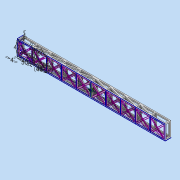
# Autodesk Inventor part: hashi1shado
Saved by Autodesk Inventor 2022 (Build 260153000, 153)
## iProperties
Created: 2024-05-14
Part Number: hashi1shado
Material: 一般
Document SubType Name: Modeling
Designer: ktamu
Density: 1 g/cm^3
Appearance: 既定
Mass: 75.4631 g
Surface Area: 713.328 cm^2
Volume: 75.4631 cm^3
Author: ktamu
Autodesk Inventor part; units mm, degrees
ref_plane "YZ Plane" through (0, 0, 0) normal (1, 0, 0) x (0, 1, 0)
ref_plane "XZ Plane" through (0, 0, 0) normal (0, 1, 0) x (-1, 0, 0)
ref_plane "XY Plane" through (0, 0, 0) normal (0, 0, 1) x (1, 0, 0)
sketch "スケッチ2" plane through (0, 0, 0) normal (1, 0, 0) x (0, 1, 0)
  line L0 (25, 10) -> (-25, 10)
  line L1 (-25, 10) -> (-25, -10)
  line L2 (-25, -10) -> (25, -10)
  line L3 (25, -10) -> (25, 10)
  line L4 (25, 10) -> (-25, -10) construction
  line L5 (-25, 10) -> (25, -10) construction
  point P0 (0, 0)
  dimension "d4" = 50
  dimension "d5" = 20
  constraints: 12 end point, 2 midpoint, 2 parallel, 1 horizontal, 1 perpendicular
  measures "d4" distance of L2.end L1.end
  measures "d5" distance of L1.end L0.end
sketch "スケッチ2 outline for 押し出し2" plane through (0, 0, 0) normal (1, 0, 0) x (0, 1, 0)
  line L0 (25, 10) -> (-25, 10)
  line L1 (25, -10) -> (25, 10)
  line L2 (-25, -10) -> (25, -10)
  line L3 (-25, 10) -> (-25, -10)
extrude "押し出し2" add sketch "スケッチ2 outline for 押し出し2" along normal mid plane 500
sketch "スケッチ3" plane through (-250, -25, 10) normal (0, 0, 1) x (1, 0, 0)
  circle A0 centre (250, 25) radius 5
  dimension "d8" = 10
  constraints: 1 centre point, 1 coincident
  measures "d8" diameter of A0
sketch "スケッチ3 outline for 押し出し3" plane through (-250, -25, 10) normal (0, 0, 1) x (1, 0, 0)
  circle A0 centre (250, 25) radius 5
extrude "押し出し3" add sketch "スケッチ3 outline for 押し出し3" along normal blind 2
sketch "SCfront" plane through (-250, -25, 10) normal (0, -1, 0) x (1, 0, 0)
  line L0 (0, -20) -> (500, -20)
  line L1 (500, 0) -> (500, -20)
  line L2 (500, 0) -> (0, 0)
  line L3 (0, -20) -> (0, 0)
  line L4 (0, 0) -> (500, 0)
  line L5 (500, 0) -> (500, -20)
  line L6 (500, -20) -> (0, -20)
  line L7 (0, -20) -> (0, 0)
  line L8 (0, 0) -> (500, -20) construction
  line L9 (500, 0) -> (0, -20) construction
  line L10 (0, 0) -> (500, 0)
  line L11 (0, -20) -> (500, -20)
  line L12 (0, 0) -> (50, 0)
  line L13 (50, 0) -> (50, -20)
  line L14 (50, -20) -> (0, -20)
  line L15 (0, -20) -> (0, 0)
  line L16 (100, 0) -> (100, -20)
  line L17 (150, 0) -> (150, -20)
  line L18 (200, 0) -> (200, -20)
  line L19 (250, 0) -> (250, -20)
  line L20 (450, 0) -> (450, -20)
  line L21 (400, 0) -> (400, -20)
  line L22 (350, 0) -> (350, -20)
  line L23 (300, 0) -> (300, -20)
  line L24 (0, 0) -> (0, -20)
  line L25 (0, 0) -> (50, -20)
  line L26 (0, -20) -> (50, 0) construction
  line L27 (50, 0) -> (100, -20)
  line L28 (100, 0) -> (50, -20)
  line L29 (52, -4) -> (98, -4)
  line L30 (98, -4) -> (98, -16)
  line L31 (98, -16) -> (52, -16)
  line L32 (52, -16) -> (52, -4)
  line L33 (75, -10) -> (98, -16) construction
  line L34 (98, -4) -> (52, -16) construction
  line L35 (102, -4) -> (148, -4)
  line L36 (102, -16) -> (102, -4)
  line L37 (148, -16) -> (102, -16)
  line L38 (148, -4) -> (148, -16)
  line L39 (152, -4) -> (198, -4)
  line L40 (152, -16) -> (152, -4)
  line L41 (198, -16) -> (152, -16)
  line L42 (198, -4) -> (198, -16)
  line L43 (202, -4) -> (248, -4)
  line L44 (202, -16) -> (202, -4)
  line L45 (248, -16) -> (202, -16)
  line L46 (248, -4) -> (248, -16)
  line L47 (252, -4) -> (298, -4)
  line L48 (252, -16) -> (252, -4)
  line L49 (298, -16) -> (252, -16)
  line L50 (298, -4) -> (298, -16)
  line L51 (302, -4) -> (348, -4)
  line L52 (302, -16) -> (302, -4)
  line L53 (348, -16) -> (302, -16)
  line L54 (348, -4) -> (348, -16)
  line L55 (352, -4) -> (398, -4)
  line L56 (352, -16) -> (352, -4)
  line L57 (398, -16) -> (352, -16)
  line L58 (398, -4) -> (398, -16)
  line L59 (402, -4) -> (448, -4)
  line L60 (402, -16) -> (402, -4)
  line L61 (448, -16) -> (402, -16)
  line L62 (448, -4) -> (448, -16)
  line L63 (48, -4) -> (48, -16)
  line L64 (48, -4) -> (4, -4)
  line L65 (4, -4) -> (4, -16.342138)
  line L66 (4, -16.342138) -> (48, -16.342138)
  line L67 (48, -16.342138) -> (48, -4)
  line L68 (452, -4) -> (452, -16)
  line L69 (452, -4) -> (496, -4)
  line L70 (496, -4) -> (496, -16.342138)
  line L71 (496, -16.342138) -> (452, -16.342138)
  line L72 (11.405237, -4) -> (48, -14.264946)
  line L73 (4, -6.077192) -> (40.594763, -16.342138)
  line L74 (488.594763, -4) -> (452, -14.264946)
  line L75 (496, -6.077192) -> (459.405237, -16.342138)
  line L76 (52, -4) -> (75, -10)
  line L77 (52, -6.066933) -> (90.076757, -16)
  line L78 (52.504844, -2.064765) -> (52.665247, -2.10661)
  line L79 (59.923243, -4) -> (98, -13.933067)
  line L80 (109.923243, -4) -> (148, -13.933067)
  line L81 (102, -6.066933) -> (140.076757, -16)
  line L82 (159.923243, -4) -> (198, -13.933067)
  line L83 (152, -6.066933) -> (190.076757, -16)
  line L84 (209.923243, -4) -> (248, -13.933067)
  line L85 (202, -6.066933) -> (240.076757, -16)
  line L86 (448, -6.066933) -> (409.923243, -16)
  line L87 (440.076757, -4) -> (402, -13.933067)
  line L88 (390.076757, -4) -> (352, -13.933067)
  line L89 (398, -6.066933) -> (359.923243, -16)
  line L90 (340.076757, -4) -> (302, -13.933067)
  line L91 (348, -6.066933) -> (309.923243, -16)
  line L92 (290.076757, -4) -> (252, -13.933067)
  line L93 (298, -6.066933) -> (259.923243, -16)
  point P0 (250, -10)
  point P1 (440.076757, -4)
  point P2 (390.076757, -4)
  point P3 (340.076757, -4)
  point P4 (290.076757, -4)
  point P5 (209.923243, -4)
  point P6 (159.923243, -4)
  point P7 (109.923243, -4)
  point P8 (60.14392, -4.057568)
  point P9 (60, -4)
  point P10 (90, -16)
  point P11 (89.85608, -15.942432)
  point P12 (48, -14.264946)
  dimension "d12" = 50
  dimension "d15" = 50
  dimension "d20" = 46
  dimension "d21" = 12
  dimension "d24" = 50
  dimension "d29" = 4
  dimension "d30" = 4
  dimension "d33" = 4
  dimension "d37" = 2
  dimension "d40" = 50
  constraints: 174 end point, 33 symmetric about line, 11 parallel, 11 point on line, 7 horizontal, 5 midpoint, 4 perpendicular, 1 vertical, 86 other
  measures "d12" distance of L13.end L14.end
  measures "d15" distance of L12.end L16.start
  measures "d20" distance of L30.end L31.end
  measures "d21" distance of L29.end L30.end
  measures "d24" distance of L29.start L35.start
  measures "d29" distance between parallel lines of L32 L63
  measures "d30" distance between parallel lines of L65 L3
  measures "d33" distance between parallel lines of L12 L64
  measures "d37" distance between parallel lines of L76 L77
  measures "d40" distance of L79.start L80.start
sketch "SCfront outline for 押し出し4" plane through (-250, -25, 10) normal (0, -1, 0) x (1, 0, 0)
  line L0 (496, -6.077192) -> (459.405237, -16.342138)
  line L1 (496, -16.342138) -> (496, -6.077192)
  line L2 (459.405237, -16.342138) -> (496, -16.342138)
  line L3 (452, -14.264946) -> (488.594763, -4)
  line L4 (452, -4) -> (452, -14.264946)
  line L5 (488.594763, -4) -> (452, -4)
  line L6 (448, -6.066933) -> (409.923243, -16)
  line L7 (448, -16) -> (448, -6.066933)
  line L8 (409.923243, -16) -> (448, -16)
  line L9 (402, -13.933067) -> (440.076757, -4)
  line L10 (402, -4) -> (402, -13.933067)
  line L11 (440.076757, -4) -> (402, -4)
  line L12 (398, -6.066933) -> (359.923243, -16)
  line L13 (398, -16) -> (398, -6.066933)
  line L14 (359.923243, -16) -> (398, -16)
  line L15 (352, -13.933067) -> (390.076757, -4)
  line L16 (352, -4) -> (352, -13.933067)
  line L17 (390.076757, -4) -> (352, -4)
  line L18 (348, -6.066933) -> (309.923243, -16)
  line L19 (348, -16) -> (348, -6.066933)
  line L20 (309.923243, -16) -> (348, -16)
  line L21 (302, -13.933067) -> (340.076757, -4)
  line L22 (302, -4) -> (302, -13.933067)
  line L23 (340.076757, -4) -> (302, -4)
  line L24 (298, -6.066933) -> (259.923243, -16)
  line L25 (298, -16) -> (298, -6.066933)
  line L26 (259.923243, -16) -> (298, -16)
  line L27 (252, -13.933067) -> (290.076757, -4)
  line L28 (252, -4) -> (252, -13.933067)
  line L29 (290.076757, -4) -> (252, -4)
  line L30 (209.923243, -4) -> (248, -13.933067)
  line L31 (248, -4) -> (209.923243, -4)
  line L32 (248, -13.933067) -> (248, -4)
  line L33 (240.076757, -16) -> (202, -6.066933)
  line L34 (202, -16) -> (240.076757, -16)
  line L35 (202, -6.066933) -> (202, -16)
  line L36 (159.923243, -4) -> (198, -13.933067)
  line L37 (198, -4) -> (159.923243, -4)
  line L38 (198, -13.933067) -> (198, -4)
  line L39 (190.076757, -16) -> (152, -6.066933)
  line L40 (152, -16) -> (190.076757, -16)
  line L41 (152, -6.066933) -> (152, -16)
  line L42 (109.923243, -4) -> (148, -13.933067)
  line L43 (148, -4) -> (109.923243, -4)
  line L44 (148, -13.933067) -> (148, -4)
  line L45 (140.076757, -16) -> (102, -6.066933)
  line L46 (102, -16) -> (140.076757, -16)
  line L47 (102, -6.066933) -> (102, -16)
  line L48 (60.14392, -4.057568) -> (98, -13.933067)
  line L49 (60, -4) -> (60.14392, -4.057568)
  line L50 (98, -4) -> (60, -4)
  line L51 (98, -13.933067) -> (98, -4)
  line L52 (89.85608, -15.942432) -> (52, -6.066933)
  line L53 (90, -16) -> (89.85608, -15.942432)
  line L54 (52, -16) -> (90, -16)
  line L55 (52, -6.066933) -> (52, -16)
  line L56 (11.405237, -4) -> (48, -14.264946)
  line L57 (48, -4) -> (11.405237, -4)
  line L58 (48, -14.264946) -> (48, -4)
  line L59 (40.594763, -16.342138) -> (4, -6.077192)
  line L60 (4, -16.342138) -> (40.594763, -16.342138)
  line L61 (4, -6.077192) -> (4, -16.342138)
extrude "押し出し4" cut sketch "SCfront outline for 押し出し4" against normal through all
sketch "SCLeft" plane through (-250, 0, 0) normal (-1, 0, 0) x (0, 0, 1)
  line L0 (10, 25) -> (10, -25)
  line L1 (-10, 25) -> (10, 25)
  line L2 (10, 25) -> (10, -25)
  line L3 (10, -25) -> (-10, -25)
  line L4 (-10, -25) -> (-10, 25)
  line L5 (-10, 25) -> (10, -25) construction
  line L6 (10, 25) -> (-10, -25) construction
  line L7 (-6, 21) -> (6, 21)
  line L8 (6, 21) -> (6, -21)
  line L9 (6, -21) -> (-6, -21)
  line L10 (-6, -21) -> (-6, 21)
  line L11 (-6, 21) -> (-1.040016, 3.640055) construction
  line L12 (6, 21) -> (-6, -21) construction
  line L13 (7.415352, 0) -> (4.34275, 0)
  line L14 (2.080031, 0) -> (6, -13.71989)
  line L15 (-3.919969, 21) -> (0, 7.28011)
  line L16 (-6, 21) -> (-1.040016, 3.640055)
  line L17 (1.040016, -3.640055) -> (6, -21)
  line L18 (-6, 13.71989) -> (-2.080031, 0)
  line L19 (0, -7.28011) -> (3.919969, -21)
  line L20 (0, 7.28011) -> (3.919969, 21)
  line L21 (-6, -13.71989) -> (-2.080031, 0)
  line L22 (-3.919969, -21) -> (0, -7.28011)
  line L23 (2.080031, 0) -> (6, 13.71989)
  line L24 (10, -25) -> (-10, -25)
  line L25 (-10, -25) -> (-10, 25)
  line L26 (-10, 25) -> (10, 25)
  line L27 (10, 25) -> (10, -25)
  line L28 (6, 15) -> (-6, 15)
  line L29 (-6, 15) -> (-6, -15)
  line L30 (-6, -15) -> (6, -15)
  line L31 (6, -15) -> (6, 15)
  line L32 (6, 15) -> (-6, -15) construction
  line L33 (-6, 15) -> (6, -15) construction
  point P0 (0, 0)
  dimension "d47" = 12
  dimension "d48" = 42
  dimension "d96" = 4
  dimension "d97" = 4
  constraints: 58 end point, 10 parallel, 6 point on line, 5 midpoint, 4 horizontal, 4 symmetric about line, 3 perpendicular
  measures "d47" distance of L8.end L9.end
  measures "d48" distance of L7.end L8.end
  measures "d96" distance between parallel lines of L4 L29
  measures "d97" distance between parallel lines of L26 L7
sketch "SCLeft outline for 押し出し5left" plane through (-250, 0, 0) normal (-1, 0, 0) x (0, 0, 1)
  line L0 (-6, 21) -> (-6, -21)
  line L1 (6, 21) -> (-6, 21)
  line L2 (6, -21) -> (6, 21)
  line L3 (-6, -21) -> (6, -21)
extrude "押し出し5left" cut sketch "SCLeft outline for 押し出し5left" against normal through all
sketch "SCLeft outline for 押し出し6" plane through (-250, 0, 0) normal (-1, 0, 0) x (0, 0, 1)
  line L0 (2.080031, 0) -> (6, 13.71989)
  line L1 (6, -13.71989) -> (2.080031, 0)
  line L2 (6, -21) -> (6, -13.71989)
  line L3 (3.919969, -21) -> (6, -21)
  line L4 (0, -7.28011) -> (3.919969, -21)
  line L5 (-3.919969, -21) -> (0, -7.28011)
  line L6 (-6, -21) -> (-3.919969, -21)
  line L7 (-6, -13.71989) -> (-6, -21)
  line L8 (-2.080031, 0) -> (-6, -13.71989)
  line L9 (-6, 13.71989) -> (-2.080031, 0)
  line L10 (-6, 21) -> (-6, 13.71989)
  line L11 (-3.919969, 21) -> (-6, 21)
  line L12 (0, 7.28011) -> (-3.919969, 21)
  line L13 (3.919969, 21) -> (0, 7.28011)
  line L14 (6, 21) -> (3.919969, 21)
  line L15 (6, 13.71989) -> (6, 21)
extrude "押し出し6" add sketch "SCLeft outline for 押し出し6" against normal blind 4
mirror "ミラー1" about plane through (0, 0, 0) normal (1, 0, 0) of "押し出し6"
sketch "SCtop" plane through (-250, -25, 10) normal (0, 0, 1) x (1, 0, 0)
  circle A0 centre (250, 25) radius 5
  line L0 (500, 0) -> (0, 0)
  line L1 (500, 50) -> (500, 0)
  line L2 (0, 50) -> (500, 50)
  line L3 (0, 0) -> (0, 50)
  circle A1 centre (250, 25) radius 5
  line L4 (0, 0) -> (0, 50)
  line L5 (0, 50) -> (500, 0) construction
  line L6 (0, 0) -> (500, 0)
  line L7 (500, 50) -> (0, 0) construction
  line L8 (0, 50) -> (500, 50)
  line L9 (500, 50) -> (500, 0)
  line L10 (500, 0) -> (0, 0)
  line L11 (0, 0) -> (0, 50)
  line L12 (0, 50) -> (500, 0) construction
  line L13 (500, 50) -> (0, 0) construction
  line L14 (0, 50) -> (500, 50)
  line L15 (0, 50) -> (50, 50)
  line L16 (50, 50) -> (50, 0)
  line L17 (50, 0) -> (0, 0)
  line L18 (0, 0) -> (0, 50)
  line L19 (100, 50) -> (100, 0)
  line L20 (150, 50) -> (150, 0)
  line L21 (200, 50) -> (200, 0)
  line L22 (250, 50) -> (250, 0)
  line L23 (300, 50) -> (300, 0)
  line L24 (350, 50) -> (350, 0)
  line L25 (400, 50) -> (400, 0)
  line L26 (450, 50) -> (450, 0)
  line L27 (50, 50) -> (100, 0)
  line L28 (0, 50) -> (50, 0)
  line L29 (50, 50) -> (0, 0)
  line L30 (98, 4) -> (60.14392, 4)
  line L31 (52, 46) -> (98, 46)
  line L32 (98, 46) -> (98, 4)
  line L33 (98, 4) -> (52, 4)
  line L34 (52, 4) -> (52, 46)
  line L35 (4, 46) -> (48, 46)
  line L36 (48, 46) -> (48, 4)
  line L37 (48, 4) -> (4, 4)
  line L38 (4, 4) -> (4, 46)
  line L39 (6.828427, 46) -> (48.025843, 4.802584)
  line L40 (4, 43.171573) -> (43.171573, 4)
  line L41 (25, 25) -> (25, 18.621886)
  line L42 (98, 0) -> (98, 4)
  line L43 (53.475936, 44.652406) -> (98, 4)
  line L44 (52, 43.291755) -> (95.033826, 4)
  line L45 (54.966174, 46) -> (98, 6.708245)
  line L46 (98, 43.291755) -> (54.966174, 4)
  line L47 (92.274678, 40.772532) -> (53.475936, 5.347594)
  line L48 (95.033826, 46) -> (52, 6.708245)
  line L49 (50.144939, 5.014494) -> (50, 4.882159)
  line L50 (73.584326, 23.584326) -> (90.909091, 40.909091)
  line L51 (92.274678, 40.772532) -> (73.516913, 23.645877) construction
  line L52 (53.475936, 5.347594) -> (52, 4) construction
  line L53 (52, 46) -> (53.475936, 44.652406) construction
  line L54 (73.516913, 26.354123) -> (98, 4) construction
  line L55 (48, 46) -> (4, 4)
  line L56 (45.103446, 46) -> (4, 6.764892)
  line L57 (48, 43.235108) -> (6.896554, 4)
  line L58 (104.966174, 46) -> (148, 6.708245)
  line L59 (145.033826, 46) -> (102, 6.708245)
  line L60 (148, 43.291755) -> (104.966174, 4)
  line L61 (102, 43.291755) -> (145.033826, 4)
  line L62 (148, 46) -> (148, 4)
  line L63 (102, 46) -> (148, 46)
  line L64 (102, 4) -> (102, 46)
  line L65 (148, 4) -> (102, 4)
  line L66 (154.966174, 46) -> (198, 6.708245)
  line L67 (195.033826, 46) -> (152, 6.708245)
  line L68 (198, 43.291755) -> (154.966174, 4)
  line L69 (152, 43.291755) -> (195.033826, 4)
  line L70 (198, 46) -> (198, 4)
  line L71 (152, 46) -> (198, 46)
  line L72 (152, 4) -> (152, 46)
  line L73 (198, 4) -> (152, 4)
  line L74 (204.966174, 46) -> (248, 6.708245)
  line L75 (245.033826, 46) -> (202, 6.708245)
  line L76 (248, 43.291755) -> (204.966174, 4)
  line L77 (202, 43.291755) -> (245.033826, 4)
  line L78 (248, 46) -> (248, 4)
  line L79 (202, 46) -> (248, 46)
  line L80 (202, 4) -> (202, 46)
  line L81 (248, 4) -> (202, 4)
  line L82 (254.966174, 46) -> (298, 6.708245)
  line L83 (295.033826, 46) -> (252, 6.708245)
  line L84 (298, 43.291755) -> (254.966174, 4)
  line L85 (252, 43.291755) -> (295.033826, 4)
  line L86 (298, 46) -> (298, 4)
  line L87 (252, 46) -> (298, 46)
  line L88 (252, 4) -> (252, 46)
  line L89 (298, 4) -> (252, 4)
  line L90 (304.966174, 46) -> (348, 6.708245)
  line L91 (345.033826, 46) -> (302, 6.708245)
  line L92 (348, 43.291755) -> (304.966174, 4)
  line L93 (302, 43.291755) -> (345.033826, 4)
  line L94 (348, 46) -> (348, 4)
  line L95 (302, 46) -> (348, 46)
  line L96 (302, 4) -> (302, 46)
  line L97 (348, 4) -> (302, 4)
  line L98 (354.966174, 46) -> (398, 6.708245)
  line L99 (395.033826, 46) -> (352, 6.708245)
  line L100 (398, 43.291755) -> (354.966174, 4)
  line L101 (352, 43.291755) -> (395.033826, 4)
  line L102 (398, 46) -> (398, 4)
  line L103 (352, 46) -> (398, 46)
  line L104 (352, 4) -> (352, 46)
  line L105 (398, 4) -> (352, 4)
  line L106 (404.966174, 46) -> (448, 6.708245)
  line L107 (445.033826, 46) -> (402, 6.708245)
  line L108 (448, 43.291755) -> (404.966174, 4)
  line L109 (402, 43.291755) -> (445.033826, 4)
  line L110 (448, 46) -> (448, 4)
  line L111 (402, 46) -> (448, 46)
  line L112 (402, 4) -> (402, 46)
  line L113 (448, 4) -> (402, 4)
  line L114 (496, 46) -> (452, 46)
  line L115 (452, 46) -> (452, 4)
  line L116 (452, 4) -> (496, 4)
  line L117 (496, 4) -> (496, 46)
  line L118 (493.171573, 46) -> (451.974157, 4.802584)
  line L119 (496, 43.171573) -> (456.828427, 4)
  line L120 (454.896554, 46) -> (496, 6.764892)
  line L121 (452, 43.235108) -> (493.103446, 4)
  point P0 (75, 25)
  point P1 (123.516913, 26.354123)
  point P2 (123.584326, 23.584326)
  point P3 (123.516913, 23.645877)
  point P4 (173.516913, 26.354123)
  point P5 (173.584326, 23.584326)
  point P6 (173.516913, 23.645877)
  point P7 (223.516913, 26.354123)
  point P8 (223.584326, 23.584326)
  point P9 (223.516913, 23.645877)
  point P10 (273.516913, 26.354123)
  point P11 (273.584326, 23.584326)
  point P12 (273.516913, 23.645877)
  point P13 (323.516913, 26.354123)
  point P14 (323.584326, 23.584326)
  point P15 (323.516913, 23.645877)
  point P16 (373.516913, 26.354123)
  point P17 (373.584326, 23.584326)
  point P18 (373.516913, 23.645877)
  point P19 (423.516913, 26.354123)
  point P20 (423.584326, 23.584326)
  point P21 (423.516913, 23.645877)
  point P22 (474.544134, 21.715707)
  point P23 (477.373326, 24.544899)
  point P24 (474.479122, 27.307549)
  point P25 (452, 4.828427)
  point P26 (471.64993, 24.478357)
  point P27 (427.966174, 25)
  point P28 (425, 22.291755)
  point P29 (425, 27.708245)
  point P30 (375, 22.291755)
  point P31 (375, 27.708245)
  point P32 (422.033826, 25)
  point P33 (377.966174, 25)
  point P34 (372.033826, 25)
  point P35 (327.966174, 25)
  point P36 (325, 22.291755)
  point P37 (325, 27.708245)
  point P38 (322.033826, 25)
  point P39 (275, 22.291755)
  point P40 (277.966174, 25)
  point P41 (275, 27.708245)
  point P42 (252, 20.417424)
  point P43 (272.033826, 25)
  point P44 (252, 29.582576)
  point P45 (225, 22.291755)
  point P46 (248, 29.582576)
  point P47 (227.966174, 25)
  point P48 (248, 20.417424)
  point P49 (225, 27.708245)
  point P50 (222.033826, 25)
  point P51 (175, 22.291755)
  point P52 (177.966174, 25)
  point P53 (175, 27.708245)
  point P54 (172.033826, 25)
  point P55 (125, 22.291755)
  point P56 (127.966174, 25)
  point P57 (125, 27.708245)
  point P58 (122.033826, 25)
  point P59 (77.966174, 25)
  point P60 (75, 22.291755)
  point P61 (75, 27.708245)
  point P62 (72.033826, 25)
  point P63 (25.455866, 21.715707)
  point P64 (28.35007, 24.478357)
  point P65 (48, 4.828427)
  point P66 (22.626674, 24.544899)
  point P67 (25.520878, 27.307549)
  point P68 (76.483087, 26.354123)
  point P69 (75, 25)
  point P70 (75, 25)
  point P71 (75, 25)
  point P72 (75, 25)
  point P73 (75, 25)
  point P74 (75, 25)
  point P75 (96, 4)
  point P76 (73.516913, 23.645877)
  point P77 (73.516913, 26.354123)
  point P78 (73.584326, 26.415674)
  point P79 (76.415674, 26.415674)
  point P80 (76.483087, 23.645877)
  point P81 (76.415674, 23.584326)
  dimension "d55" = 50
  dimension "d56" = 50
  dimension "d59" = 50
  dimension "d64" = 46
  dimension "d65" = 42
  dimension "d66" = 44
  dimension "d67" = 42
  dimension "d68" = 4
  dimension "d69" = 4
  dimension "d76" = 2
  dimension "d77" = 2
  dimension "d80" = 50
  constraints: 226 end point, 97 point on line, 20 midpoint, 17 parallel, 12 symmetric about line, 6 horizontal, 5 perpendicular, 1 vertical, 185 other
  measures "d55" distance of L16.end L17.end
  measures "d56" distance of L15.end L16.end
  measures "d59" distance of L15.end L19.start
  measures "d64" distance of L30.start L33.end
  measures "d65" distance of L31.end L30.start
  measures "d66" distance of L36.end L37.end
  measures "d67" distance of L35.end L36.end
  measures "d68" distance between parallel lines of L2 L35
  measures "d69" distance between parallel lines of L34 L36
  measures "d76" distance between parallel lines of L55 L56
  measures "d77" distance between parallel lines of L55 L57
  measures "d80" distance of L45.start L58.start
sketch "SCtop outline for 押し出し7" plane through (-250, -25, 10) normal (0, 0, 1) x (1, 0, 0)
  line L0 (456.828427, 4) -> (493.103446, 4)
  line L1 (474.544134, 21.715707) -> (456.828427, 4)
  line L2 (493.103446, 4) -> (474.544134, 21.715707)
  line L3 (496, 6.764892) -> (496, 43.171573)
  line L4 (477.373326, 24.544899) -> (496, 6.764892)
  line L5 (496, 43.171573) -> (477.373326, 24.544899)
  line L6 (493.171573, 46) -> (454.896554, 46)
  line L7 (474.479122, 27.307549) -> (493.171573, 46)
  line L8 (454.896554, 46) -> (474.479122, 27.307549)
  line L9 (452, 43.235108) -> (452, 4.828427)
  line L10 (471.64993, 24.478357) -> (452, 43.235108)
  line L11 (452, 4.828427) -> (471.64993, 24.478357)
  line L12 (448, 6.708245) -> (448, 43.291755)
  line L13 (427.966174, 25) -> (448, 6.708245)
  line L14 (448, 43.291755) -> (427.966174, 25)
  line L15 (404.966174, 4) -> (445.033826, 4)
  line L16 (425, 22.291755) -> (404.966174, 4)
  line L17 (445.033826, 4) -> (425, 22.291755)
  line L18 (445.033826, 46) -> (404.966174, 46)
  line L19 (425, 27.708245) -> (445.033826, 46)
  line L20 (404.966174, 46) -> (425, 27.708245)
  line L21 (354.966174, 4) -> (395.033826, 4)
  line L22 (375, 22.291755) -> (354.966174, 4)
  line L23 (395.033826, 4) -> (375, 22.291755)
  line L24 (395.033826, 46) -> (354.966174, 46)
  line L25 (375, 27.708245) -> (395.033826, 46)
  line L26 (354.966174, 46) -> (375, 27.708245)
  line L27 (402, 43.291755) -> (402, 6.708245)
  line L28 (422.033826, 25) -> (402, 43.291755)
  line L29 (402, 6.708245) -> (422.033826, 25)
  line L30 (398, 6.708245) -> (398, 43.291755)
  line L31 (377.966174, 25) -> (398, 6.708245)
  line L32 (398, 43.291755) -> (377.966174, 25)
  line L33 (352, 43.291755) -> (352, 6.708245)
  line L34 (372.033826, 25) -> (352, 43.291755)
  line L35 (352, 6.708245) -> (372.033826, 25)
  line L36 (348, 6.708245) -> (348, 43.291755)
  line L37 (327.966174, 25) -> (348, 6.708245)
  line L38 (348, 43.291755) -> (327.966174, 25)
  line L39 (304.966174, 4) -> (345.033826, 4)
  line L40 (325, 22.291755) -> (304.966174, 4)
  line L41 (345.033826, 4) -> (325, 22.291755)
  line L42 (345.033826, 46) -> (304.966174, 46)
  line L43 (325, 27.708245) -> (345.033826, 46)
  line L44 (304.966174, 46) -> (325, 27.708245)
  line L45 (302, 43.291755) -> (302, 6.708245)
  line L46 (322.033826, 25) -> (302, 43.291755)
  line L47 (302, 6.708245) -> (322.033826, 25)
  line L48 (254.966174, 4) -> (295.033826, 4)
  line L49 (275, 22.291755) -> (254.966174, 4)
  line L50 (295.033826, 4) -> (275, 22.291755)
  line L51 (298, 6.708245) -> (298, 43.291755)
  line L52 (277.966174, 25) -> (298, 6.708245)
  line L53 (298, 43.291755) -> (277.966174, 25)
  line L54 (295.033826, 46) -> (254.966174, 46)
  line L55 (275, 27.708245) -> (295.033826, 46)
  line L56 (254.966174, 46) -> (275, 27.708245)
  line L57 (252, 20.417424) -> (252, 6.708245)
  arc A0 (252, 29.582576) -> (252, 20.417424) centre (250, 25) cw
  line L58 (252, 43.291755) -> (252, 29.582576)
  line L59 (272.033826, 25) -> (252, 43.291755)
  line L60 (252, 6.708245) -> (272.033826, 25)
  line L61 (204.966174, 4) -> (245.033826, 4)
  line L62 (225, 22.291755) -> (204.966174, 4)
  line L63 (245.033826, 4) -> (225, 22.291755)
  line L64 (248, 29.582576) -> (248, 43.291755)
  arc A1 (248, 20.417424) -> (248, 29.582576) centre (250, 25) cw
  line L65 (248, 6.708245) -> (248, 20.417424)
  line L66 (227.966174, 25) -> (248, 6.708245)
  line L67 (248, 43.291755) -> (227.966174, 25)
  line L68 (245.033826, 46) -> (204.966174, 46)
  line L69 (225, 27.708245) -> (245.033826, 46)
  line L70 (204.966174, 46) -> (225, 27.708245)
  line L71 (202, 43.291755) -> (202, 6.708245)
  line L72 (222.033826, 25) -> (202, 43.291755)
  line L73 (202, 6.708245) -> (222.033826, 25)
  line L74 (154.966174, 4) -> (195.033826, 4)
  line L75 (175, 22.291755) -> (154.966174, 4)
  line L76 (195.033826, 4) -> (175, 22.291755)
  line L77 (198, 6.708245) -> (198, 43.291755)
  line L78 (177.966174, 25) -> (198, 6.708245)
  line L79 (198, 43.291755) -> (177.966174, 25)
  line L80 (195.033826, 46) -> (154.966174, 46)
  line L81 (175, 27.708245) -> (195.033826, 46)
  line L82 (154.966174, 46) -> (175, 27.708245)
  line L83 (152, 43.291755) -> (152, 6.708245)
  line L84 (172.033826, 25) -> (152, 43.291755)
  line L85 (152, 6.708245) -> (172.033826, 25)
  line L86 (104.966174, 4) -> (145.033826, 4)
  line L87 (125, 22.291755) -> (104.966174, 4)
  line L88 (145.033826, 4) -> (125, 22.291755)
  line L89 (148, 6.708245) -> (148, 43.291755)
  line L90 (127.966174, 25) -> (148, 6.708245)
  line L91 (148, 43.291755) -> (127.966174, 25)
  line L92 (145.033826, 46) -> (104.966174, 46)
  line L93 (125, 27.708245) -> (145.033826, 46)
  line L94 (104.966174, 46) -> (125, 27.708245)
  line L95 (102, 43.291755) -> (102, 6.708245)
  line L96 (122.033826, 25) -> (102, 43.291755)
  line L97 (102, 6.708245) -> (122.033826, 25)
  line L98 (98, 43.291755) -> (77.966174, 25)
  line L99 (98, 6.708245) -> (98, 43.291755)
  line L100 (77.966174, 25) -> (98, 6.708245)
  line L101 (75, 22.291755) -> (54.966174, 4)
  line L102 (54.966174, 4) -> (95.033826, 4)
  line L103 (95.033826, 4) -> (75, 22.291755)
  line L104 (75, 27.708245) -> (95.033826, 46)
  line L105 (54.966174, 46) -> (75, 27.708245)
  line L106 (95.033826, 46) -> (54.966174, 46)
  line L107 (52, 6.708245) -> (72.033826, 25)
  line L108 (52, 43.291755) -> (52, 6.708245)
  line L109 (72.033826, 25) -> (52, 43.291755)
  line L110 (25.455866, 21.715707) -> (6.896554, 4)
  line L111 (43.171573, 4) -> (25.455866, 21.715707)
  line L112 (6.896554, 4) -> (43.171573, 4)
  line L113 (48, 43.235108) -> (28.35007, 24.478357)
  line L114 (48, 4.828427) -> (48, 43.235108)
  line L115 (28.35007, 24.478357) -> (48, 4.828427)
  line L116 (4, 6.764892) -> (22.626674, 24.544899)
  line L117 (4, 43.171573) -> (4, 6.764892)
  line L118 (22.626674, 24.544899) -> (4, 43.171573)
  line L119 (25.520878, 27.307549) -> (45.103446, 46)
  line L120 (6.828427, 46) -> (25.520878, 27.307549)
  line L121 (45.103446, 46) -> (6.828427, 46)
extrude "押し出し7" cut sketch "SCtop outline for 押し出し7" against normal through all
sketch "スケッチ7" plane through (0, 0, 12) normal (0, 0, 1) x (1, 0, 0)
  line L0 (-2, 21) -> (-2, -21)
  line L1 (2, -18.291755) -> (2, -4.582576)
  line L2 (2, -21) -> (2, 21)
  circle A0 centre (0, 0) radius 5
  arc A1 (-2, -4.582576) -> (2, -4.582576) centre (0, 0) ccw
  line L3 (-2, -4.582576) -> (-2, 4.582576)
  line L4 (2, -4.582576) -> (2, 4.582576)
  circle A2 centre (0, 0) radius 1
  point P0 (-2, -4.582576)
  dimension "d89" = 2
  constraints: 4 end point, 2 point on circle, 2 point on line, 1 centre point, 1 coincident
  measures "d89" diameter of A2
sketch "スケッチ7 outline for 押し出し8" plane through (0, 0, 12) normal (0, 0, 1) x (1, 0, 0)
  arc A0 (2, -4.582576) -> (2, 4.582576) centre (0, 0) ccw
  line L0 (2, 4.582576) -> (2, -4.582576)
  arc A1 (-2, 4.582576) -> (-2, -4.582576) centre (0, 0) ccw
  line L1 (-2, -4.582576) -> (-2, 4.582576)
extrude "押し出し8" cut sketch "スケッチ7 outline for 押し出し8" against normal through all
sketch "スケッチ7 outline for 押し出し9" plane through (0, 0, 12) normal (0, 0, 1) x (1, 0, 0)
  arc A0 (-2, -4.582576) -> (2, -4.582576) centre (0, 0) ccw
  line L0 (-2, 4.582576) -> (-2, -4.582576)
  line L1 (2, -4.582576) -> (2, 4.582576)
  arc A1 (2, 4.582576) -> (-2, 4.582576) centre (0, 0) ccw
  circle A2 centre (0, 0) radius 1
extrude "押し出し9" cut sketch "スケッチ7 outline for 押し出し9" against normal blind 2
sketch "スケッチ7 outline for 押し出し10" plane through (0, 0, 12) normal (0, 0, 1) x (1, 0, 0)
  circle A0 centre (0, 0) radius 1
extrude "押し出し10" cut sketch "スケッチ7 outline for 押し出し10" against normal blind 1
sketch "スケッチ7 outline for 押し出し11" plane through (0, 0, 12) normal (0, 0, 1) x (1, 0, 0)
  circle A0 centre (0, 0) radius 1
extrude "押し出し11" cut sketch "スケッチ7 outline for 押し出し11" against normal blind 2
sketch "SCLeft outline for 押し出し12" plane through (-250, 0, 0) normal (-1, 0, 0) x (0, 0, 1)
  line L0 (6, -21) -> (6, -13.71989)
  line L1 (3.919969, -21) -> (6, -21)
  line L2 (0, -7.28011) -> (3.919969, -21)
  line L3 (-3.919969, -21) -> (0, -7.28011)
  line L4 (-6, -21) -> (-3.919969, -21)
  line L5 (-6, -13.71989) -> (-6, -21)
  line L6 (-2.080031, 0) -> (-6, -13.71989)
  line L7 (-6, 13.71989) -> (-2.080031, 0)
  line L8 (-6, 21) -> (-6, 13.71989)
  line L9 (-3.919969, 21) -> (-6, 21)
  line L10 (0, 7.28011) -> (-3.919969, 21)
  line L11 (3.919969, 21) -> (0, 7.28011)
  line L12 (6, 21) -> (3.919969, 21)
  line L13 (6, 13.71989) -> (6, 21)
  line L14 (2.080031, 0) -> (6, 13.71989)
  line L15 (6, -13.71989) -> (2.080031, 0)
extrude "押し出し12" cut sketch "SCLeft outline for 押し出し12" against normal through all
sketch "SCtop outline for 押し出し13" plane through (-250, -25, 10) normal (0, 0, 1) x (1, 0, 0)
  line L0 (45.103446, 46) -> (25.520878, 27.307549)
  line L1 (48, 46) -> (45.103446, 46)
  line L2 (48, 43.235108) -> (48, 46)
  line L3 (28.35007, 24.478357) -> (48, 43.235108)
  line L4 (48, 4.828427) -> (28.35007, 24.478357)
  line L5 (48, 4) -> (48, 4.828427)
  line L6 (43.171573, 4) -> (48, 4)
  line L7 (25.455866, 21.715707) -> (43.171573, 4)
  line L8 (6.896554, 4) -> (25.455866, 21.715707)
  line L9 (4, 4) -> (6.896554, 4)
  line L10 (4, 6.764892) -> (4, 4)
  line L11 (22.626674, 24.544899) -> (4, 6.764892)
  line L12 (4, 43.171573) -> (22.626674, 24.544899)
  line L13 (4, 46) -> (4, 43.171573)
  line L14 (6.828427, 46) -> (4, 46)
  line L15 (25.520878, 27.307549) -> (6.828427, 46)
  line L16 (452, 46) -> (452, 43.235108)
  line L17 (454.896554, 46) -> (452, 46)
  line L18 (474.479122, 27.307549) -> (454.896554, 46)
  line L19 (493.171573, 46) -> (474.479122, 27.307549)
  line L20 (496, 46) -> (493.171573, 46)
  line L21 (496, 43.171573) -> (496, 46)
  line L22 (477.373326, 24.544899) -> (496, 43.171573)
  line L23 (496, 6.764892) -> (477.373326, 24.544899)
  line L24 (496, 4) -> (496, 6.764892)
  line L25 (493.103446, 4) -> (496, 4)
  line L26 (474.544134, 21.715707) -> (493.103446, 4)
  line L27 (456.828427, 4) -> (474.544134, 21.715707)
  line L28 (452, 4) -> (456.828427, 4)
  line L29 (452, 4.828427) -> (452, 4)
  line L30 (471.64993, 24.478357) -> (452, 4.828427)
  line L31 (452, 43.235108) -> (471.64993, 24.478357)
extrude "押し出し13" cut sketch "SCtop outline for 押し出し13" against normal through all
sketch "SCtop outline for 押し出し14" plane through (-250, -25, 10) normal (0, 0, 1) x (1, 0, 0)
  line L0 (448, 46) -> (402, 46)
  line L1 (448, 43.291755) -> (448, 46)
  line L2 (427.966174, 25) -> (448, 43.291755)
  line L3 (448, 6.708245) -> (427.966174, 25)
  line L4 (448, 4) -> (448, 6.708245)
  line L5 (445.033826, 4) -> (448, 4)
  line L6 (425, 22.291755) -> (445.033826, 4)
  line L7 (404.966174, 4) -> (425, 22.291755)
  line L8 (402, 4) -> (404.966174, 4)
  line L9 (402, 6.708245) -> (402, 4)
  line L10 (422.033826, 25) -> (402, 6.708245)
  line L11 (402, 43.291755) -> (422.033826, 25)
  line L12 (402, 46) -> (402, 43.291755)
  line L13 (96, 4) -> (75, 25)
  line L14 (95.033826, 4) -> (96, 4)
  line L15 (75, 22.291755) -> (95.033826, 4)
  line L16 (54.966174, 4) -> (75, 22.291755)
  line L17 (52, 4) -> (54.966174, 4)
  line L18 (52, 6.708245) -> (52, 4)
  line L19 (72.033826, 25) -> (52, 6.708245)
  line L20 (52, 43.291755) -> (72.033826, 25)
  line L21 (52, 46) -> (52, 43.291755)
  line L22 (54.966174, 46) -> (52, 46)
  line L23 (75, 27.708245) -> (54.966174, 46)
  line L24 (95.033826, 46) -> (75, 27.708245)
  line L25 (98, 46) -> (95.033826, 46)
  line L26 (98, 43.291755) -> (98, 46)
  line L27 (77.966174, 25) -> (98, 43.291755)
  line L28 (98, 6.708245) -> (77.966174, 25)
  line L29 (98, 4) -> (98, 6.708245)
  line L30 (75, 25) -> (98, 4)
  line L31 (73.516913, 23.645877) -> (75, 25)
  line L32 (73.584326, 23.584326) -> (73.516913, 23.645877)
  line L33 (75, 25) -> (73.584326, 23.584326)
  line L34 (73.584326, 26.415674) -> (75, 25)
  line L35 (73.516913, 26.354123) -> (73.584326, 26.415674)
  line L36 (75, 25) -> (73.516913, 26.354123)
  line L37 (76.483087, 26.354123) -> (75, 25)
  line L38 (76.415674, 26.415674) -> (76.483087, 26.354123)
  line L39 (75, 25) -> (76.415674, 26.415674)
extrude "押し出し14" cut sketch "SCtop outline for 押し出し14" against normal through all
sketch "sideRemover1" plane through (-250, -25, -10) normal (0, -1, 0) x (1, 0, 0)
  line L0 (496, 3.657862) -> (459.405237, 3.657862)
  line L1 (488.594763, 16) -> (452, 16)
  line L2 (496, 3.657862) -> (452, 3.657862)
  line L3 (452, 3.657862) -> (452, 16)
  line L4 (452, 16) -> (496, 16)
  line L5 (496, 16) -> (496, 3.657862)
  line L6 (4, 13.922808) -> (4, 3.657862)
  line L7 (48, 5.735054) -> (48, 16)
  line L8 (4, 3.657862) -> (48, 3.657862)
  line L9 (48, 3.657862) -> (48, 16)
  line L10 (48, 16) -> (4, 16)
  line L11 (4, 16) -> (4, 3.657862)
  line L12 (0, 16) -> (4, 16)
  line L13 (48, 3.657862) -> (4, 3.657862)
  line L14 (4, 3.657862) -> (4, 16)
  line L15 (4, 16) -> (48, 16)
  line L16 (48, 16) -> (48, 3.657862)
  point P0 (250, 10)
  constraints: 24 end point, 6 parallel, 3 horizontal, 3 perpendicular
sketch "sideRemover1 outline for 押し出し15" plane through (-250, -25, -10) normal (0, -1, 0) x (1, 0, 0)
  line L0 (4, 16) -> (4, 13.922808)
  line L1 (48, 16) -> (4, 16)
  line L2 (48, 5.735054) -> (48, 16)
  line L3 (48, 3.657862) -> (48, 5.735054)
  line L4 (4, 3.657862) -> (48, 3.657862)
  line L5 (4, 13.922808) -> (4, 3.657862)
extrude "押し出し15" cut sketch "sideRemover1 outline for 押し出し15" against normal through all
sketch "スケッチ9" plane through (-250, -25, -10) normal (0, -1, 0) x (1, 0, 0)
  line L0 (488.594763, 16) -> (452, 16)
  line L1 (459.405237, 3.657862) -> (496, 3.657862)
  line L2 (452, 16) -> (496, 16)
  line L3 (496, 16) -> (496, 3.657862)
  line L4 (496, 3.657862) -> (452, 3.657862)
  line L5 (452, 3.657862) -> (452, 16)
  point P0 (250, 10)
  constraints: 8 end point, 2 parallel, 1 horizontal, 1 perpendicular
sketch "スケッチ9 outline for 押し出し16" plane through (-250, -25, -10) normal (0, -1, 0) x (1, 0, 0)
  line L0 (496, 3.657862) -> (496, 16)
  line L1 (459.405237, 3.657862) -> (496, 3.657862)
  line L2 (452, 3.657862) -> (459.405237, 3.657862)
  line L3 (452, 16) -> (452, 3.657862)
  line L4 (488.594763, 16) -> (452, 16)
  line L5 (496, 16) -> (488.594763, 16)
extrude "押し出し16" cut sketch "スケッチ9 outline for 押し出し16" against normal through all
sketch "SCtop outline for 押し出し17" plane through (-250, -25, 10) normal (0, 0, 1) x (1, 0, 0)
  line L0 (76.483087, 23.645877) -> (76.415674, 23.584326)
  line L1 (98, 4) -> (76.483087, 23.645877)
  line L2 (96, 4) -> (98, 4)
  line L3 (76.415674, 23.584326) -> (96, 4)
extrude "押し出し17" cut sketch "SCtop outline for 押し出し17" against normal through all
sketch "SCtop outline for 押し出し18" plane through (-250, -25, 10) normal (0, 0, 1) x (1, 0, 0)
  line L0 (152, 46) -> (152, 43.291755)
  line L1 (154.966174, 46) -> (152, 46)
  line L2 (175, 27.708245) -> (154.966174, 46)
  line L3 (195.033826, 46) -> (175, 27.708245)
  line L4 (198, 46) -> (195.033826, 46)
  line L5 (198, 43.291755) -> (198, 46)
  line L6 (177.966174, 25) -> (198, 43.291755)
  line L7 (198, 6.708245) -> (177.966174, 25)
  line L8 (198, 4) -> (198, 6.708245)
  line L9 (195.033826, 4) -> (198, 4)
  line L10 (175, 22.291755) -> (195.033826, 4)
  line L11 (154.966174, 4) -> (175, 22.291755)
  line L12 (152, 4) -> (154.966174, 4)
  line L13 (152, 6.708245) -> (152, 4)
  line L14 (172.033826, 25) -> (152, 6.708245)
  line L15 (152, 43.291755) -> (172.033826, 25)
  line L16 (345.033826, 4) -> (348, 4)
  line L17 (325, 22.291755) -> (345.033826, 4)
  line L18 (304.966174, 4) -> (325, 22.291755)
  line L19 (302, 4) -> (304.966174, 4)
  line L20 (302, 6.708245) -> (302, 4)
  line L21 (322.033826, 25) -> (302, 6.708245)
  line L22 (302, 43.291755) -> (322.033826, 25)
  line L23 (302, 46) -> (302, 43.291755)
  line L24 (304.966174, 46) -> (302, 46)
  line L25 (325, 27.708245) -> (304.966174, 46)
  line L26 (345.033826, 46) -> (325, 27.708245)
  line L27 (348, 46) -> (345.033826, 46)
  line L28 (348, 43.291755) -> (348, 46)
  line L29 (327.966174, 25) -> (348, 43.291755)
  line L30 (348, 6.708245) -> (327.966174, 25)
  line L31 (348, 4) -> (348, 6.708245)
  line L32 (352, 46) -> (352, 43.291755)
  line L33 (354.966174, 46) -> (352, 46)
  line L34 (375, 27.708245) -> (354.966174, 46)
  line L35 (395.033826, 46) -> (375, 27.708245)
  line L36 (398, 46) -> (395.033826, 46)
  line L37 (398, 43.291755) -> (398, 46)
  line L38 (377.966174, 25) -> (398, 43.291755)
  line L39 (398, 6.708245) -> (377.966174, 25)
  line L40 (398, 4) -> (398, 6.708245)
  line L41 (395.033826, 4) -> (398, 4)
  line L42 (375, 22.291755) -> (395.033826, 4)
  line L43 (354.966174, 4) -> (375, 22.291755)
  line L44 (352, 4) -> (354.966174, 4)
  line L45 (352, 6.708245) -> (352, 4)
  line L46 (372.033826, 25) -> (352, 6.708245)
  line L47 (352, 43.291755) -> (372.033826, 25)
  line L48 (102, 46) -> (102, 43.291755)
  line L49 (104.966174, 46) -> (102, 46)
  line L50 (125, 27.708245) -> (104.966174, 46)
  line L51 (145.033826, 46) -> (125, 27.708245)
  line L52 (148, 46) -> (145.033826, 46)
  line L53 (148, 43.291755) -> (148, 46)
  line L54 (127.966174, 25) -> (148, 43.291755)
  line L55 (148, 6.708245) -> (127.966174, 25)
  line L56 (148, 4) -> (148, 6.708245)
  line L57 (145.033826, 4) -> (148, 4)
  line L58 (125, 22.291755) -> (145.033826, 4)
  line L59 (104.966174, 4) -> (125, 22.291755)
  line L60 (102, 4) -> (104.966174, 4)
  line L61 (102, 6.708245) -> (102, 4)
  line L62 (122.033826, 25) -> (102, 6.708245)
  line L63 (102, 43.291755) -> (122.033826, 25)
extrude "押し出し18" cut sketch "SCtop outline for 押し出し18" against normal blind 4
sketch "スケッチ10" plane through (-250, -25, 10) normal (0, 0, 1) x (1, 0, 0)
  line L0 (402, 4) -> (402, 46)
  line L1 (402, 46) -> (448, 46)
  line L2 (448, 46) -> (448, 4)
  line L3 (448, 4) -> (402, 4)
  line L4 (98, 4) -> (52, 4)
  line L5 (52, 4) -> (52, 46)
  line L6 (52, 46) -> (98, 46)
  line L7 (98, 46) -> (98, 4)
  line L8 (252, 6.708245) -> (252, 43.291755)
  line L9 (252, 43.291755) -> (272.033826, 25)
  line L10 (272.033826, 25) -> (252, 6.708245)
  line L11 (248, 43.291755) -> (248, 6.708245)
  line L12 (248, 6.708245) -> (227.966174, 25)
  line L13 (227.966174, 25) -> (248, 43.291755)
  line L14 (48, 4) -> (4, 4)
  line L15 (4, 4) -> (4, 46)
  line L16 (4, 46) -> (48, 46)
  line L17 (48, 46) -> (48, 4)
  line L18 (298, 6.708245) -> (277.966174, 25)
  line L19 (277.966174, 25) -> (298, 43.291755)
  line L20 (298, 43.291755) -> (298, 6.708245)
  line L21 (295.033826, 46) -> (275, 27.708245)
  line L22 (275, 27.708245) -> (254.966174, 46)
  line L23 (254.966174, 46) -> (295.033826, 46)
  line L24 (245.033826, 46) -> (225, 27.708245)
  line L25 (225, 27.708245) -> (204.966174, 46)
  line L26 (204.966174, 46) -> (245.033826, 46)
  line L27 (204.966174, 4) -> (225, 22.291755)
  line L28 (225, 22.291755) -> (245.033826, 4)
  line L29 (245.033826, 4) -> (204.966174, 4)
  line L30 (254.966174, 4) -> (275, 22.291755)
  line L31 (275, 22.291755) -> (295.033826, 4)
  line L32 (295.033826, 4) -> (254.966174, 4)
  line L33 (302, 4) -> (302, 46)
  line L34 (302, 46) -> (348, 46)
  line L35 (348, 46) -> (348, 4)
  line L36 (348, 4) -> (302, 4)
  line L37 (496, 46) -> (496, 4)
  line L38 (496, 4) -> (452, 4)
  line L39 (452, 4) -> (452, 46)
  line L40 (452, 46) -> (496, 46)
  line L41 (202, 43.291755) -> (222.033826, 25)
  line L42 (222.033826, 25) -> (202, 6.708245)
  line L43 (202, 6.708245) -> (202, 43.291755)
  line L44 (500, 0) -> (0, 0)
  line L45 (500, 50) -> (500, 0)
  line L46 (0, 50) -> (500, 50)
  line L47 (0, 0) -> (0, 50)
  line L48 (148, 46) -> (148, 4)
  line L49 (148, 4) -> (102, 4)
  line L50 (102, 4) -> (102, 46)
  line L51 (102, 46) -> (148, 46)
  line L52 (198, 46) -> (198, 4)
  line L53 (198, 4) -> (152, 4)
  line L54 (152, 4) -> (152, 46)
  line L55 (152, 46) -> (198, 46)
  line L56 (398, 46) -> (398, 4)
  line L57 (398, 4) -> (352, 4)
  line L58 (352, 4) -> (352, 46)
  line L59 (352, 46) -> (398, 46)
  line L60 (448, 4) -> (448, 46)
  line L61 (452, 4) -> (496, 4)
  line L62 (448, 46) -> (452, 46)
  line L63 (452, 46) -> (452, 4)
  line L64 (452, 4) -> (448, 4)
  line L65 (448, 4) -> (448, 46)
  line L66 (4, 46) -> (48, 46)
  line L67 (52, 4) -> (52, 46)
  line L68 (48, 46) -> (52, 46)
  line L69 (52, 46) -> (52, 4)
  line L70 (52, 4) -> (48, 4)
  line L71 (48, 4) -> (48, 46)
  point P0 (250, 25)
  point P1 (448, 4)
  constraints: 16 end point, 4 parallel, 2 horizontal, 2 perpendicular
sketch "スケッチ10 outline for 押し出し19" plane through (-250, -25, 10) normal (0, 0, 1) x (1, 0, 0)
  line L0 (48, 4) -> (52, 4)
  line L1 (48, 46) -> (48, 4)
  line L2 (52, 46) -> (48, 46)
  line L3 (52, 4) -> (52, 46)
  line L4 (452, 46) -> (448, 46)
  line L5 (452, 4) -> (452, 46)
  line L6 (448, 4) -> (452, 4)
  line L7 (448, 46) -> (448, 4)
extrude "押し出し19" cut sketch "スケッチ10 outline for 押し出し19" against normal blind 4
sketch "SCtop outline for 押し出し20" plane through (-250, -25, 10) normal (0, 0, 1) x (1, 0, 0)
  line L0 (76.415674, 26.415674) -> (75, 25)
  line L1 (76.483087, 26.354123) -> (76.415674, 26.415674)
  line L2 (75, 25) -> (76.483087, 26.354123)
  line L3 (73.584326, 26.415674) -> (73.516913, 26.354123)
  line L4 (75, 25) -> (73.584326, 26.415674)
  line L5 (73.516913, 26.354123) -> (75, 25)
  line L6 (73.584326, 23.584326) -> (75, 25)
  line L7 (73.516913, 23.645877) -> (73.584326, 23.584326)
  line L8 (75, 25) -> (73.516913, 23.645877)
  line L9 (76.415674, 23.584326) -> (76.483087, 23.645877)
  line L10 (75, 25) -> (76.415674, 23.584326)
  line L11 (76.483087, 23.645877) -> (75, 25)
extrude "押し出し20" cut sketch "SCtop outline for 押し出し20" against normal through all
